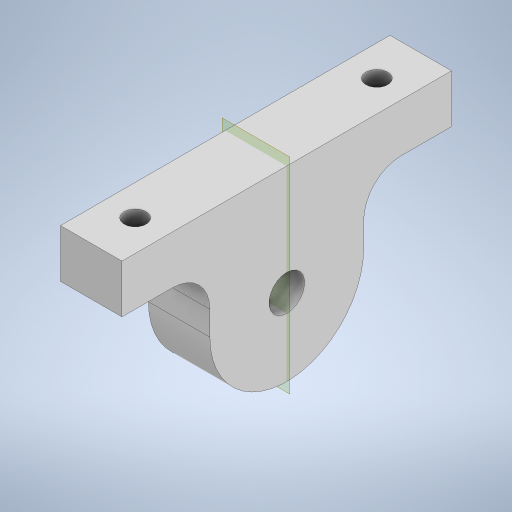
# Autodesk Inventor part: Passive Wheel 8mm bore bracket
Saved by Autodesk Inventor 2024 (Build 280153020, 153B)
## iProperties
Created: 2024-02-16
Part Number: Passive Wheel 8mm bore bracket
Material: Generic
Document SubType Name: Modeling
Designer: scottst
Density: 1 g/cm^3
Appearance: Default
Author: scottst
Autodesk Inventor part; units mm, degrees
ref_plane "YZ Plane" through (0, 0, 0) normal (1, 0, 0) x (0, 1, 0)
ref_plane "XZ Plane" through (0, 0, 0) normal (0, 1, 0) x (-1, 0, 0)
ref_plane "XY Plane" through (0, 0, 0) normal (0, 0, 1) x (1, 0, 0)
sketch "Sketch1" plane through (0, 0, 0) normal (1, 0, 0) x (0, 1, 0)
  circle A0 centre (0, 0) radius 4.05
  circle A1 centre (0, 0) radius 17.5
  line L0 (0, 17.5) -> (25, 17.5)
  line L1 (0, -17.5) -> (25, -17.5)
  line L2 (25, -17.5) -> (25, 17.5)
  dimension "d0" = 8.1
  dimension "d1" = 35
  dimension "d2" = 25
  dimension "d3" = 25
  constraints: 6 end point, 2 centre point, 2 coincident, 2 horizontal, 2 point on circle, 1 perpendicular, 1 tangent
  measures "d0" diameter of A0
  measures "d1" diameter of A1
  measures "d2" distance of L0.start L0.end
  measures "d3" distance of L1.start L1.end
extrude "Extrusion1" add sketch "Sketch1" along normal blind 14
ref_plane "Work Plane1" through (0, 0, 0) normal (0, 0, -1) x (-1, 0, 0)
sketch "Sketch2" plane through (14, 0, 0) normal (1, 0, 0) x (0, 0, -1)
  line L0 (17.5, 25) -> (-17.5, 25) projected
  line L1 (17.5, 25) -> (37.5, 25)
  line L2 (37.5, 25) -> (37.5, 14)
  line L3 (37.5, 14) -> (17.5, 14)
  line L4 (17.5, 14) -> (17.5, 25)
  point P0 (0, 0)
  dimension "d6" = 20
  dimension "d7" = 11
  constraints: 8 end point, 2 parallel, 1 horizontal, 1 perpendicular
  measures "d6" distance of L2.end L3.end
  measures "d7" distance of L1.end L2.end
extrude "Extrusion2" add sketch "Sketch2" against normal blind 14
fillet "Fillet1" radius 8.5 1 edges at (7, 14, -17.5)
sketch "Sketch3" plane through (0, 14, -37.5) normal (0, -1, 0) x (1, 0, 0)
  line L0 (14, 0) -> (0, 0) construction
  line L1 (7, 0) -> (7, 10) construction
  point P0 (0, 37.5)
  dimension "d11" = 10
  constraints: 2 end point, 1 coincident, 1 midpoint, 1 vertical
  measures "d11" distance of L1.start L1.end
hole "Hole1" at (7, 14, -27.5) direction (0, 1, 0) diameter 5 end through all countersink diameter 9.5 countersink angle 90
sketch "Sketch4" plane through (0, 14, -37.5) normal (0, -1, 0) x (1, 0, 0)
  arc A0 (2.4931, 11.5) -> (11.5069, 11.5) centre (7, 10) ccw projected
  circle A1 centre (7, 10) radius 4.75
  point P0 (0, 37.5)
  point P1 (11.5069, 11.5)
  constraints: 1 centre point, 1 coincident, 1 concentric
extrude "Extrusion3" cut sketch "Sketch4" along normal blind 14
mirror "Mirror1" about plane through (0, 0, 0) normal (0, 0, -1) of "Hole1", "Extrusion3", "Extrusion2", "Fillet1"
body "Solid1"
